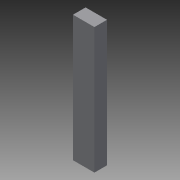
# Autodesk Inventor part: CNC-Z-axis- linear drawer slider
Saved by Autodesk Inventor 2015 (Build 190159000, 159)
## iProperties
Created: 2015-03-21
Part Number: CNC-Z-axis- linear drawer slider
Material: Generic
Document SubType Name: Modeling
Designer: Bangladesh
Density: 1 g/cm^3
Appearance: Default
Author: Bangladesh
Autodesk Inventor part; units mm, degrees
ref_plane "YZ Plane" through (0, 0, 0) normal (1, 0, 0) x (0, 1, 0)
ref_plane "XZ Plane" through (0, 0, 0) normal (0, 1, 0) x (-1, 0, 0)
ref_plane "XY Plane" through (0, 0, 0) normal (0, 0, 1) x (1, 0, 0)
sketch "Sketch2" plane through (0, 0, 0) normal (0, 0, 1) x (1, 0, 0)
  line L0 (-21.59, 127) -> (21.59, 127)
  line L1 (21.59, 127) -> (21.59, -127)
  line L2 (21.59, -127) -> (-21.59, -127)
  line L3 (-21.59, -127) -> (-21.59, 127)
  line L4 (-21.59, 127) -> (21.59, -127) construction
  line L5 (21.59, 127) -> (-21.59, -127) construction
  point P0 (0, 0)
  dimension "d0" = 43.18
  dimension "d1" = 254
  constraints: 12 end point, 2 midpoint, 2 parallel, 1 horizontal, 1 perpendicular
  measures "d0" distance of L1.end L2.end
  measures "d1" distance of L0.end L1.end
extrude "Extrusion1" add sketch "Sketch2" along normal mid plane 25.4
body "Solid1"
